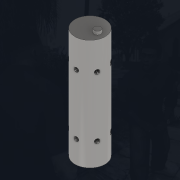
# Autodesk Inventor part: Grip Base
Saved by Autodesk Inventor 2021 (Build 250183000, 183)
## iProperties
Created: 2021-01-08
Part Number: Grip Base
Material: Generic
Document SubType Name: Modeling
Designer: Alex
Density: 1 g/cm^3
Appearance: Default
Mass: 62.8276 g
Surface Area: 110.145 cm^2
Volume: 62.8276 cm^3
Author: Alex
Autodesk Inventor part; units mm, degrees
ref_plane "YZ Plane" through (0, 0, 0) normal (1, 0, 0) x (0, 1, 0)
sketch "Sketch1" plane through (0, 0, 0) normal (0, 1, 0) x (-1, 0, 0)
  circle A0 centre (0, 0) radius 14
  dimension "d0" = 28
  constraints: 1 centre point, 1 coincident
  measures "d0" diameter of A0
extrude "Extrusion1" add sketch "Sketch1" along normal blind 100
ref_plane "Work Plane1" through (0, 91.9, 0) normal (0, 1, 0) x (1, 0, 0)
sketch "Sketch2" plane through (0, 91.9, 0) normal (0, 1, 0) x (1, 0, 0)
  arc A0 (-4.9212, -15.749) -> (7.4582, -14.7182) centre (0, 0) ccw
  line L0 (-4.9212, -15.749) -> (7.4582, -14.7182)
  line L1 (3.8609, -16.2352) -> (3.7603, -15.0261)
  line L2 (1.2685, -15.2336) -> (-1.2229, -15.4411)
  line L3 (-1.1222, -16.6505) -> (-1.2229, -15.4411)
  line L4 (1.7436, -20.9268) -> (4.2347, -20.7192)
  line L5 (4.2347, -20.7192) -> (3.8609, -16.2352)
  line L6 (-1.1222, -16.6505) -> (-0.7484, -21.1346)
  line L7 (-0.7484, -21.1346) -> (1.7436, -20.9268)
  line L8 (8.9092, -10.799) -> (11.1788, -12.1357)
  arc A1 (11.1788, -12.1357) -> (16.4755, -0.8993) centre (0, 0.0004) ccw
  line L9 (11.1788, -12.1357) -> (16.4755, -0.8993)
  line L10 (11.1788, -12.1357) -> (12.7611, -8.7789)
  line L11 (12.7611, -8.7789) -> (17.9297, -11.2153)
  line L12 (17.9297, -11.2153) -> (20.0617, -6.6927)
  line L13 (20.0617, -6.6927) -> (14.893, -4.2562)
  arc A2 (16.0997, 3.6126) -> (9.0172, 13.8181) centre (0, 0) ccw
  line L14 (16.0997, 3.6126) -> (9.0172, 13.8181)
  line L15 (16.0997, 3.6126) -> (13.9839, 6.6614)
  line L16 (13.9839, 6.6614) -> (18.6782, 9.9192)
  line L17 (18.6782, 9.9192) -> (15.8275, 14.0269)
  line L18 (15.8275, 14.0269) -> (11.1332, 10.7691)
  arc A3 (4.9196, 15.7499) -> (-7.4587, 14.7181) centre (0.0003, 0.0003) ccw
  line L19 (4.9196, 15.7499) -> (-7.4587, 14.7181)
  line L20 (4.9196, 15.7499) -> (1.2214, 15.4417)
  line L21 (1.2214, 15.4417) -> (0.7467, 21.1359)
  line L22 (0.7467, 21.1359) -> (-4.236, 20.7206)
  line L23 (-4.236, 20.7206) -> (-3.7613, 15.0263)
  arc A4 (-11.1784, 12.1373) -> (-16.4754, 0.901) centre (0, 0.0009) ccw
  line L24 (-14, 0) -> (-16.4754, 0.901)
  line L25 (-11.1784, 12.1373) -> (-16.4754, 0.901)
  line L26 (-11.1784, 12.1373) -> (-12.7608, 8.7805)
  line L27 (-12.7608, 8.7805) -> (-17.9293, 11.2171)
  line L28 (-17.9293, 11.2171) -> (-20.0613, 6.6944)
  line L29 (-20.0613, 6.6944) -> (-14.8929, 4.2579)
  arc A5 (-16.0997, -3.6126) -> (-9.0172, -13.8181) centre (0, 0) ccw
  line L30 (-9.0172, -13.8181) -> (-16.0997, -3.6126)
  line L31 (-16.0997, -3.6126) -> (-13.9839, -6.6614)
  line L32 (-13.9839, -6.6614) -> (-18.6782, -9.9192)
  line L33 (-18.6782, -9.9192) -> (-15.8275, -14.0269)
  line L34 (-15.8275, -14.0269) -> (-11.1332, -10.7691)
  line L35 (11.1788, -12.1357) -> (-16.4754, 0.901)
  line L36 (16.4755, -0.8993) -> (-11.1784, 12.1373)
  line L37 (-9.0172, -13.8181) -> (16.0997, 3.6126)
  line L38 (-16.0997, -3.6126) -> (9.0172, 13.8181)
  line L39 (-4.9212, -15.749) -> (-7.4587, 14.7181)
  line L40 (7.4582, -14.7182) -> (4.9196, 15.7499)
  line L41 (5.0265, 14.4675) -> (-7.3518, 13.4357)
  dimension "d4" = 2.5
  dimension "d5" = 3.711
  dimension "d6" = 5.714
  dimension "d7" = 5
  dimension "d8" = 3.711
  dimension "d9" = 5.714
  dimension "d10" = 5
  dimension "d11" = 3.711
  dimension "d12" = 5.714
  dimension "d13" = 5
  dimension "d14" = 3.711
  dimension "d15" = 5.714
  dimension "d16" = 5
  dimension "d17" = 3.711
  dimension "d18" = 5.714
  dimension "d19" = 5
  dimension "d20" = 5.258
  dimension "d21" = 0.001
  dimension "d22" = 5.0004
  dimension "d23" = 5.0004
  dimension "d24" = 36.2862
  dimension "d25" = 12.3632
  constraints: 84 end point, 20 perpendicular, 13 point on line, 12 point on circle, 6 centre point, 4 parallel, 1 midpoint
  measures "d4" distance of L2.start L2.end
  measures "d5" distance of L8.end L10.end
  measures "d6" distance of L10.end L11.end
  measures "d7" distance of L11.end L13.start
  measures "d8" distance of L14.start L15.end
  measures "d9" distance of L15.end L16.end
  measures "d10" distance of L16.end L18.start
  measures "d11" distance of L20.start L20.end
  measures "d12" distance of L20.end L21.end
  measures "d13" distance of L21.end L22.end
  measures "d14" distance of L26.start L26.end
  measures "d15" distance of L26.end L27.end
  measures "d16" distance of L27.end L28.end
  measures "d17" distance of L31.start L32.start
  measures "d18" distance of L32.start L33.start
  measures "d19" distance of L33.start L34.start
  measures "d20" angle of L8 L11
  measures "d21" distance between parallel lines of L5 L21
  measures "d22" distance between parallel lines of L5 L6
  measures "d23" distance between parallel lines of L1 L3
  measures "d24" distance between parallel lines of L20 L7
  measures "d25" distance from line of L7.end L8
ref_plane "Work Plane2" through (5.0265, 91.9, -14.4675) normal (-0.0831, 0, -0.9965) x (-0.9965, 0, 0.0831)
sketch "Sketch3" plane through (5.0265, 91.9, -14.4675) normal (-0.0831, 0, -0.9965) x (-0.9965, 0, 0.0831)
  line L0 (0, 0) -> (12.421, 0)
  line L1 (20.2109, -91.9) -> (-7.7891, -91.9) projected
  line L2 (0, -91.9) -> (12.421, -91.9)
  line L3 (12.421, 0) -> (12.421, -91.9) construction
  line L4 (6.2105, 0) -> (6.2105, -15) construction
  circle A0 centre (6.2105, -15) radius 2
  line L5 (6.2105, -91.9) -> (6.2105, -76.9) construction
  circle A1 centre (6.2105, -76.9) radius 2
  point P0 (6.2109, -91.9)
  dimension "d27" = 12.421
  dimension "d28" = 15
  dimension "d29" = 4
  dimension "d30" = 15
  dimension "d31" = 4
  constraints: 10 end point, 2 centre point, 2 coincident, 2 midpoint, 1 horizontal, 1 perpendicular, 1 point on line
  measures "d27" distance of L0.start L0.end
  measures "d28" distance of L4.start L4.end
  measures "d29" diameter of A0
  measures "d30" distance of L5.start L5.end
  measures "d31" diameter of A1
ref_plane "Work Plane3" through (4.9434, 91.9, -15.4641) normal (-0.0831, 0, -0.9965) x (-0.9965, 0, 0.0831)
sketch "Sketch4" plane through (4.9434, 91.9, -15.4641) normal (-0.0831, 0, -0.9965) x (-0.9965, 0, 0.0831)
  line L0 (0, 0) -> (12.421, 0)
  line L1 (16.664, -85.9) -> (-11.336, -85.9)
  line L2 (-3.5469, -85.9) -> (12.421, -85.9)
  line L3 (12.421, 0) -> (12.421, -85.9) construction
  line L4 (6.2105, 0) -> (6.2105, -15) construction
  circle A0 centre (6.2105, -15) radius 2
  line L5 (6.2105, -85.9) -> (6.2105, -70.9) construction
  circle A1 centre (6.2105, -70.9) radius 2
  line L6 (6.2105, -76.9) -> (6.2105, -70.9) construction
  point P0 (6.2109, -91.9)
  point P1 (6.2109, -91.9)
  dimension "d33" = 12.421
  dimension "d34" = 15
  dimension "d35" = 4
  dimension "d36" = 15
  dimension "d37" = 4
  dimension "d43" = 6
  constraints: 12 end point, 2 centre point, 2 coincident, 2 vertical, 1 horizontal, 1 midpoint, 1 point on line, 4 other
  measures "d33" distance of L0.start L0.end
  measures "d34" distance of L4.start L4.end
  measures "d35" diameter of A0
  measures "d36" distance of L5.start L5.end
  measures "d37" diameter of A1
  measures "d43" distance of L6.start L6.end
extrude "Extrusion2" cut sketch "Sketch4" against normal blind 5.5
pattern_circular "Circular Pattern1" count 6 over 360 about axis through (0, -10, 0) along (0, 1, 0) of "Extrusion2"
sketch "Sketch5" plane through (0, 100, 0) normal (0, 1, 0) x (1, 0, 0)
  line L0 (0, 0) -> (14, 0) construction
  circle A0 centre (0, 0) radius 14 construction
  line L1 (0, 0) -> (7, 0) construction
  circle A1 centre (7, 0) radius 3
  dimension "d44" = 6
  constraints: 4 end point, 1 centre point, 1 coincident, 1 horizontal, 1 horizontal alignment, 1 midpoint, 1 other
  measures "d44" diameter of A1
extrude "Extrusion3" add sketch "Sketch5" along normal blind 6
sketch "Sketch6" plane through (0, 100, 0) normal (0, 1, 0) x (1, 0, 0)
  circle A0 centre (0, 0) radius 14
  constraints: 1 centre point, 1 coincident
extrude "Extrusion4" add sketch "Sketch6" along normal blind 3
body "Solid1"
